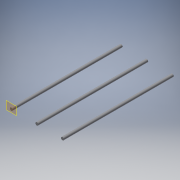
# Autodesk Inventor part: Y rails
Saved by Autodesk Inventor 2016 (Build 200138000, 138)
## iProperties
Created: 2016-04-23
Part Number: Y rails
Material: Generic
Document SubType Name: Modeling
Designer: Scott
Density: 1 g/cm^3
Appearance: Default
Author: Scott
Autodesk Inventor part; units mm, degrees
ref_plane "YZ Plane" through (0, 0, 0) normal (1, 0, 0) x (0, 1, 0)
ref_plane "XZ Plane" through (0, 0, 0) normal (0, 1, 0) x (-1, 0, 0)
ref_plane "Work Plane1" through (-140, 0, 0) normal (0, 0, 1) x (1, 0, 0)
sketch "Sketch1" plane through (-140, 0, 0) normal (0, 0, 1) x (1, 0, 0)
  circle A0 centre (0, 7.84) radius 4 projected
  circle A1 centre (140, 7.84) radius 4 projected
  circle A2 centre (70, 7.84) radius 5 projected
  circle A3 centre (70, 7.84) radius 4
  point P0 (140, 0)
  dimension "d0" = 8
  constraints: 1 centre point, 1 coincident
  measures "d0" diameter of A3
ref_plane "Work Plane2" through (-149.963, -13.75, -300.8725) normal (0, 0, -1) x (0, 1, 0)
extrude "Extrusion1" add sketch "Sketch1" against normal up to surface (300.8725 mm away) contours A0 | A1 | A3
body "Solid1"
